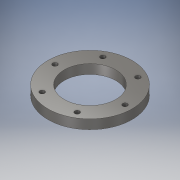
# Autodesk Inventor part: BearingRing
Saved by Autodesk Inventor 2019 (Build 230136000, 136)
## iProperties
Created: 2018-12-09
Part Number: BearingRing
Material: Aluminum 6061
Document SubType Name: Modeling
Designer: steelen
Density: 2.7 g/cm^3
Appearance: Semi-Polished
Author: steelen
Autodesk Inventor part; units mm, degrees
ref_plane "YZ Plane" through (0, 0, 0) normal (1, 0, 0) x (0, 1, 0)
ref_plane "XZ Plane" through (0, 0, 0) normal (0, 1, 0) x (-1, 0, 0)
ref_plane "XY Plane" through (0, 0, 0) normal (0, 0, 1) x (1, 0, 0)
sketch "Sketch1" plane through (0, 0, 0) normal (0, 1, 0) x (-1, 0, 0)
  circle A0 centre (0, 0) radius 35
  circle A1 centre (0, 0) radius 57.15
  dimension "d0" = 114.3
  dimension "d1" = 70
  constraints: 2 centre point, 2 coincident
  measures "d0" diameter of A1
  measures "d1" diameter of A0
extrude "Extrusion1" add sketch "Sketch1" along normal blind 12.7
sketch "Sketch2" plane through (0, 12.7, 0) normal (0, 1, 0) x (1, 0, 0)
  circle A0 centre (0, 0) radius 57.15 projected
  line L0 (-57.15, 0) -> (-47.625, 0)
  point P0 (-23.8125, 41.2445)
  point P1 (23.8125, 41.2445)
  point P2 (47.625, 0)
  point P3 (23.8125, -41.2445)
  point P4 (-23.8125, -41.2445)
  dimension "d4" = 9.525
  dimension "d7" = 360
  constraints: 2 end point, 2 horizontal, 1 horizontal alignment, 8 other
  measures "d4" distance of L0.start L0.end
hole "Hole1" at (-47.625, 12.7, 0) at (-23.8125, 12.7, -41.2445) at (23.8125, 12.7, -41.2445) at (47.625, 12.7, 0) at (23.8125, 12.7, 41.2445) at (-23.8125, 12.7, 41.2445) direction (0, -1, 0) diameter 6.5278 end through all clearance for "Socket Head Cap Screw" size "1/4" standard "Ansi Unified Screw Threads"
body "Solid1"
